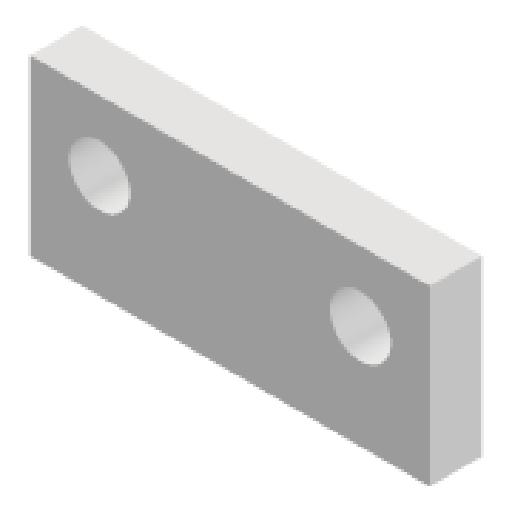
# Autodesk Inventor part: Nozzlecam_PCB_Mount
Saved by Autodesk Inventor 2023.2 (Build 272271000, 271)
## iProperties
Created: 2023-02-07
Part Number: Nozzlecam_PCB_Mount
Material: ABS Plastic
Document SubType Name: Modeling
Designer: remop
Density: 1.06 g/cm^3
Appearance: Smooth - Light Orange
Author: remop
Autodesk Inventor part; units mm, degrees
ref_plane "YZ Plane" through (0, 0, 0) normal (1, 0, 0) x (0, 1, 0)
ref_plane "XZ Plane" through (0, 0, 0) normal (0, 1, 0) x (-1, 0, 0)
ref_plane "XY Plane" through (0, 0, 0) normal (0, 0, 1) x (1, 0, 0)
sketch "Sketch1" plane through (0, 0, 0) normal (0, 0, 1) x (1, 0, 0)
  circle A0 centre (-10, 0) radius 1.75
  circle A1 centre (10, 0) radius 1.75
  line L0 (-15, 4) -> (15, 4)
  line L1 (15, 4) -> (15, -6)
  line L2 (15, -6) -> (-15, -6)
  line L3 (-15, -6) -> (-15, 4)
  point P0 (0, 0)
  dimension "d0" = 10
  dimension "d1" = 10
  dimension "d2" = 3.5
  dimension "d3" = 5
  dimension "d4" = 5
  dimension "d5" = 4
  dimension "d6" = 10
  constraints: 8 end point, 2 centre point, 2 coincident, 2 horizontal alignment, 2 parallel, 1 equal radius, 1 horizontal, 1 perpendicular
  measures "d0" distance of point (10, 0) point (0, 0)
  measures "d1" distance of point (-10, 0) point (0, 0)
  measures "d2" diameter of A1
  measures "d3" distance from line of L3 point (-10, 0)
  measures "d4" distance from line of L1 A1.centre
  measures "d5" distance from line of L0 A0.centre
  measures "d6" distance of L2.end L0.start
extrude "Extrusion1" add sketch "Sketch1" along normal blind 3
sketch "Sketch2" plane through (0, 0, 3) normal (0, 0, 1) x (1, 0, 0)
  line L0 (-15, -6) -> (15, -6) projected
  line L1 (15, -6) -> (15, 4) projected
  line L2 (15, 4) -> (-15, 4) projected
  line L3 (-15, 4) -> (-15, -6) projected
  circle A0 centre (10, 0) radius 1.75 projected
  circle A1 centre (-10, 0) radius 1.75 projected
  line L4 (15, -6) -> (15, 4) projected
  line L5 (-15, -6) -> (15, -6)
  line L6 (15, -6) -> (15, -4)
  line L7 (15, -4) -> (-15, -4)
  line L8 (-15, -4) -> (-15, -6)
  point P0 (0, 0)
  dimension "d9" = 2
  constraints: 8 end point, 2 parallel, 1 horizontal, 1 perpendicular, 1 point on line
  measures "d9" distance between parallel lines of L0 L7
extrude "Extrusion2" add sketch "Sketch2" along normal blind 20 contours L3 L7 L1 L0
sketch "Sketch4" plane through (-15, -4, 3) normal (0, 1, 0) x (1, 0, 0)
  line L0 (0, 0) -> (30, 0) projected
  line L1 (0, 0) -> (0, -20) projected
  line L2 (30, -20) -> (0, -20) projected
  line L3 (30, 0) -> (30, -20) projected
  circle A0 centre (2, -6) radius 1
  circle A1 centre (28, -6) radius 1
  circle A2 centre (28, -17) radius 1
  circle A3 centre (2, -17) radius 1
  circle A4 centre (2, -6) radius 2
  line L4 (0, 3) -> (0, -20) projected
  circle A5 centre (2, -17) radius 2
  circle A6 centre (28, -17) radius 2
  line L5 (30, 3) -> (30, -20) projected
  circle A7 centre (28, -6) radius 2
  point P0 (15, 3)
  dimension "d12" = 2
  dimension "d13" = 26
  dimension "d14" = 11
  dimension "d15" = 2
  dimension "d16" = 6
  constraints: 8 centre point, 4 coincident, 4 tangent, 3 equal radius, 2 horizontal alignment, 2 vertical alignment
  measures "d12" diameter of A0
  measures "d13" distance of A1.centre A0.centre
  measures "d14" distance of A3.centre A0.centre
  measures "d15" distance from line of L1 A0.centre
  measures "d16" distance from line of L0 A0.centre
extrude "Extrusion3" add sketch "Sketch4" along normal blind 1 contours A4 | A5 | A6 | A7
sketch "Sketch5" plane through (-13, -4, 9) normal (0, 1, 0) x (1, 0, 0)
  circle A0 centre (0, 0) radius 1 projected
  circle A1 centre (26, 0) radius 1 projected
  circle A2 centre (26, -11) radius 1 projected
  circle A3 centre (0, -11) radius 1 projected
  point P0 (13, 9)
extrude "Extrusion4" cut sketch "Sketch5" against normal through all
equation "\"d1\" = d0"
equation "\"d4\" = d3"
body "Solid1"
